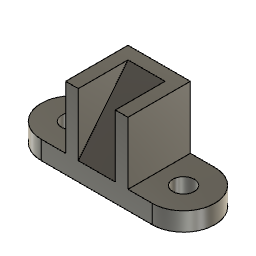
Figure A2 v1 (Autodesk Fusion 360 design; units mm, degrees)
Autodesk Fusion 360 part; units mm, degrees
note: some values were not read from the file. Set by a fixed rule: which sketch regions a step uses.
sketch "Sketch1" plane through (0, 0, 0) normal (0, 0, 1) x (1, 0, 0)
  line L0 (57, 32) -> (-57, 32)
  line L1 (-57, 32) -> (-57, -32)
  line L2 (-57, -32) -> (57, -32)
  line L3 (57, -32) -> (57, 32)
  line L4 (57, 32) -> (-57, -32) construction
  line L5 (-57, 32) -> (57, -32) construction
  circle A0 centre (-57, 0) radius 11
  circle A1 centre (-57, 0) radius 32
  circle A2 centre (57, 0) radius 11
  circle A3 centre (57, 0) radius 32
  dimension "d1" = 114
  dimension "d2" = 64
  dimension "d3" = 22
  dimension "d4" = 32
  dimension "d5" = 22
  dimension "d7" = 32
  constraint horizontal L0
  constraint perpendicular L0 L1
  constraint parallel L0 L2
  constraint parallel L1 L3
  constraint coincident L4 origin
  constraint coincident L5 origin
  constraint midpoint L1 A0.centre
  constraint concentric A0 A1
  constraint midpoint L3 A2.centre
  constraint concentric A2 A3
  measures "d1" distance of L1.end L2.end
  measures "d2" distance of L0.end L1.end
  measures "d3" diameter of A0
  measures "d4" radius of A1
  measures "d5" diameter of A2
  measures "d7" radius of A3
extrude "Extrude1" add sketch "Sketch1" along normal blind 19 contours L0 L2 A1 A3 | L3 A2 A3 | L3 A2 A3 | L1 A0 A1 | L1 A0 A1
sketch "Sketch2" plane through (0, 0, 19) normal (0, 0, 1) x (-1, 0, 0)
  circle A0 centre (-57, 0) radius 11
  circle A1 centre (57, 0) radius 11
  arc A2 (-57, 32) -> (-57, -32) centre (-57, 0) ccw
  line L0 (-57, -32) -> (57, -32)
  arc A3 (57, -32) -> (57, 32) centre (57, 0) ccw
  line L1 (57, 32) -> (-57, 32)
  line L2 (-32, -32) -> (32, -32)
  line L3 (32, -32) -> (32, 32)
  line L4 (32, 32) -> (-32, 32)
  line L5 (-32, 32) -> (-32, -32)
  line L6 (-32, -32) -> (32, 32) construction
  line L7 (32, -32) -> (-32, 32) construction
  line L8 (19, 32) -> (-19, 32)
  line L9 (-19, 32) -> (-19, -19)
  line L10 (-19, -19) -> (19, -19)
  line L11 (19, -19) -> (19, 32)
  dimension "d10" = 64
  dimension "d11" = 64
  dimension "d12" = 38
  dimension "d13" = 51
  dimension "d14" = 13
  dimension "d15" = 13
  constraint horizontal L2
  constraint perpendicular L2 L3
  constraint parallel L2 L4
  constraint parallel L3 L5
  constraint coincident L6 origin
  constraint coincident L7 origin
  constraint horizontal L8
  constraint vertical L9
  constraint horizontal L10
  constraint vertical L11
  constraint coincident L4 L8.start
  measures "d10" distance of L3.end L4.end
  measures "d11" distance of L2.end L3.end
  measures "d12" distance of L8.start L8.end
  measures "d13" distance of L8.start L10.end
  measures "d14" distance of L5 L9
  measures "d15" distance of L2 L10
extrude "Extrude2" add sketch "Sketch2" along normal blind 64 contours L0 L1 L2 L3 L4 L5 L9 L10 L11
sketch "Sketch3" plane through (19, 0, 0) normal (-1, 0, 0) x (0, -1, 0)
  line L0 (-19, 19) -> (32, 19)
  line L1 (32, 19) -> (32, 83)
  line L2 (32, 83) -> (-19, 83)
  line L3 (-19, 83) -> (-19, 19)
  line L4 (32, 19) -> (-19, 83)
  line L5 (-19, 19) -> (32, 19)
  line L6 (-19, 19) -> (-19, 83)
  constraint coincident L0.end L1.start
  constraint coincident L2.end L3.start
  constraint coincident L0.start L3.end
extrude "Extrude3" add sketch "Sketch3" along normal blind 40 contours L0 L3 L4 L5 L6
equation "d14 = ( ( 64 - 38 ) / 2 ) * 1 mm"
named bodies: "Main Part"
